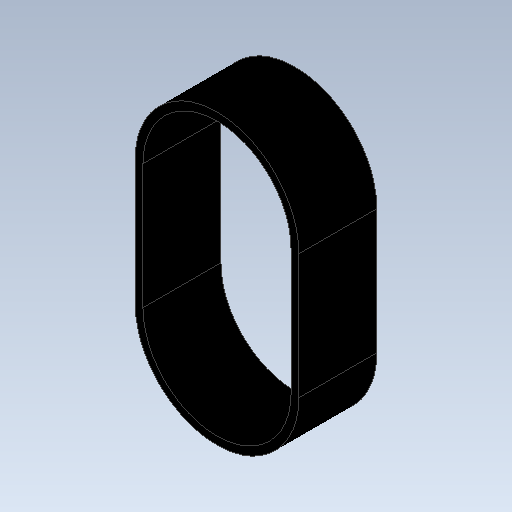
# Autodesk Inventor part: Colierî
Saved by Autodesk Inventor 2020 (Build 240168000, 168)
## iProperties
Created: 2020-12-24
Part Number: Colierî
Material: Generic
Document SubType Name: Modeling
Designer: Iulian Bors
Density: 1 g/cm^3
Appearance: Default(1)
Mass: 0.948319 g
Surface Area: 20.863 cm^2
Volume: 0.948319 cm^3
Author: Iulian Bors
Subject: wire necklace
Autodesk Inventor part; units mm, degrees
ref_plane "YZ Plane" through (0, 0, 0) normal (1, 0, 0) x (0, 1, 0)
ref_plane "XZ Plane" through (0, 0, 0) normal (0, 1, 0) x (-1, 0, 0)
ref_plane "XY Plane" through (0, 0, 0) normal (0, 0, 1) x (1, 0, 0)
sketch "Sketch1" plane through (0, 0, 0) normal (0, 0, 1) x (1, 0, 0)
  line L0 (0, 0) -> (0, 16) construction
  line L1 (-9.5, 0) -> (-9.5, 16)
  line L2 (9.5, 16) -> (9.5, 0)
  arc A0 (-9.5, 0) -> (9.5, 0) centre (0, 0) ccw
  arc A1 (9.5, 16) -> (-9.5, 16) centre (0, 16) ccw
  line L3 (-10.5, 16) -> (-10.5, 0)
  arc A2 (-10.5, 0) -> (10.5, 0) centre (0, 0) ccw
  line L4 (10.5, 0) -> (10.5, 16)
  arc A3 (10.5, 16) -> (-10.5, 16) centre (0, 16) ccw
  point P0 (0, 8)
  dimension "d3" = 9.5
  dimension "d4" = 16
  dimension "d5" = 1
  constraints: 12 end point, 8 point on circle, 4 centre point, 4 tangent, 2 parallel, 1 midpoint, 1 vertical, 3 other
  measures "d3" radius of A0
  measures "d4" distance of L0.start L0.end
  measures "d5" distance between parallel lines of L1 L3
extrude "Extrusion1" add sketch "Sketch1" along normal mid plane 10
body "Solid1"
